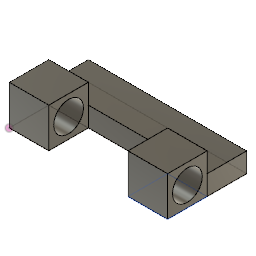
Arm Chassis Connector (Autodesk Fusion 360 design; units mm, degrees)
Autodesk Fusion 360 part; units mm, degrees
sketch "Sketch1" plane through (0, 0, 0) normal (0, 0, 1) x (1, 0, 0)
  line L0 (0, 0) -> (10, 0)
  line L1 (10, 0) -> (10, 10)
  line L2 (10, 10) -> (0, 10)
  line L3 (0, 10) -> (0, 0)
  line L4 (0, 10) -> (40, 10)
  line L5 (40, 10) -> (40, 20)
  line L6 (40, 20) -> (0, 20)
  line L7 (0, 20) -> (0, 10)
  line L8 (40, 0) -> (30, 0)
  line L9 (30, 0) -> (30, 10)
  line L10 (30, 10) -> (40, 10)
  line L11 (40, 10) -> (40, 0)
  dimension "d6" = 10
  dimension "d7" = 10
  dimension "d8" = 40
  dimension "d9" = 10
  dimension "d14" = 10
  dimension "d15" = 10
  constraint horizontal L0
  constraint vertical L1
  constraint horizontal L2
  constraint vertical L3
  constraint coincident L0.start L3.end
  constraint horizontal L4
  constraint vertical L5
  constraint horizontal L6
  constraint vertical L7
  constraint horizontal L8
  constraint vertical L9
  constraint horizontal L10
  constraint vertical L11
  measures "d6" distance of L0.start L0.end
  measures "d7" distance of L0.start L2.end
  measures "d8" distance of L2.end L4.end
  measures "d9" distance of L2.end L6.end
  measures "d14" distance of L8.start L8.end
  measures "d15" distance of L8.start L4.end
extrude "Extrude3" add sketch "Sketch1" along normal blind 10 contours L4 L8 L9 L10 L11 makes body 1
extrude "Extrude2" add sketch "Sketch1" along normal blind 5 separate body contours L2 L4 L5 L6 L7 L10 makes body 2
extrude "Extrude1" add sketch "Sketch1" along normal blind 10 separate body contours L0 L1 L2 L3 L4 makes body 3
sketch "Sketch2" plane through (40, 0, 0) normal (1, 0, 0) x (0, 1, 0)
  line L0 (0, 0) -> (10, 0)
  line L1 (10, 0) -> (10, 10)
  line L2 (10, 10) -> (0, 10)
  line L3 (0, 10) -> (0, 0)
  circle A0 centre (5, 5) radius 3.75
  dimension "d18" = 7.5
  dimension "d19" = 5
  dimension "d20" = 5
  measures "d18" diameter of A0
  measures "d19" distance of L3 A0.centre
  measures "d20" distance of L2 A0.centre
extrude "Extrude4" cut sketch "Sketch2" against normal blind 140 contours A0 bodies 1 3
equation "side = 10 mm"
equation "base_length = 40 mm"
equation "base_width = 10 mm"
equation "base_height = 5 mm"
equation "dowel_pin_hole_radius = ( 3 * side / 4 ) / 2"
equation "d6 = side"
equation "d7 = side"
equation "d8 = base_length"
equation "d9 = base_width"
equation "d10 = side"
equation "d12 = base_height"
equation "d14 = side"
equation "d15 = side"
equation "d16 = side"
equation "d18 = dowel_pin_hole_radius * 2"
equation "d19 = side / 2"
equation "d20 = side / 2"
equation "d21 = -( base_length + extra )"
equation "extra = 100 mm"
